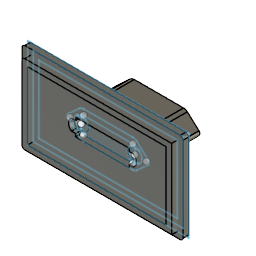
DD-fiche-v4 (Autodesk Fusion 360 design; units mm, degrees)
part number: 2025-12-20-11-26-56-309
Autodesk Fusion 360 part; units mm, degrees
note: some values were not read from the file. Set by a fixed rule: which sketch regions a step uses.
sketch "Esquisse1" plane through (0, 0, 0) normal (0, 1, 0) x (1, 0, 0)
  circle A0 centre (10, -10) radius 2.5
  line L0 (8.5, -12) -> (11.5, -12)
  line L1 (8.5, -8) -> (11.5, -8)
  circle A1 centre (29, -10) radius 2.5
  line L2 (27.5, -12) -> (30.5, -12)
  line L3 (27.5, -8) -> (30.5, -8)
  line L4 (5.3139, -10.7399) -> (9.4279, -14.4799)
  line L5 (10.7732, -15) -> (28.2268, -15)
  line L6 (29.5721, -14.4799) -> (33.6861, -10.7399)
  line L7 (33.6861, -9.2601) -> (29.5721, -5.5201)
  line L8 (28.2268, -5) -> (10.7732, -5)
  line L9 (9.4279, -5.5201) -> (5.3139, -9.2601)
  arc A2 (9.4279, -14.4799) -> (10.7732, -15) centre (10.7732, -13) ccw
  arc A3 (28.2268, -15) -> (29.5721, -14.4799) centre (28.2268, -13) ccw
  arc A4 (29.5721, -5.5201) -> (28.2268, -5) centre (28.2268, -7) ccw
  arc A5 (10.7732, -5) -> (9.4279, -5.5201) centre (10.7732, -7) ccw
  arc A6 (5.3139, -9.2601) -> (5.3139, -10.7399) centre (5.9866, -10) ccw
  arc A7 (33.6861, -10.7399) -> (33.6861, -9.2601) centre (33.0134, -10) ccw
  line L10 (-8.9501, 6) -> (48.0499, 6)
  line L11 (48.0499, 6) -> (48.0499, -26)
  line L12 (48.0499, -26) -> (-8.9501, -26)
  line L13 (-8.9501, -26) -> (-8.9501, 6)
  line L14 (-7, -24) -> (46, -24)
  line L15 (46, -24) -> (46, 4)
  line L16 (46, 4) -> (-7, 4)
  line L17 (-7, 4) -> (-7, -24)
  line L18 (-5, -22) -> (44, -22)
  line L19 (44, -22) -> (44, 2)
  line L20 (44, 2) -> (-5, 2)
  line L21 (-5, 2) -> (-5, -22)
  line L22 (10, -12) -> (8.5, -12)
  line L23 (10, -13) -> (29, -13)
  line L24 (29, -7) -> (10, -7)
  line L25 (10, -13) -> (10, -7)
  line L26 (29, -13) -> (29, -7)
  constraint coincident A0 L0.start
  constraint coincident A0 L0.end
  constraint horizontal L0
  constraint coincident A0 L1.start
  constraint coincident A0 L1.end
  constraint parallel L0 L1
  constraint coincident A1 L2.start
  constraint coincident A1 L2.end
  constraint horizontal L2
  constraint coincident A1 L3.start
  constraint coincident A1 L3.end
  constraint parallel L2 L3
  constraint horizontal L5
  constraint horizontal L8
  constraint equal A2 A3
  constraint equal A2 A4
  constraint equal A2 A5
  constraint horizontal L10
  constraint vertical L11
  constraint horizontal L12
  constraint vertical L13
  constraint horizontal L14
  constraint vertical L15
  constraint horizontal L16
  constraint vertical L17
  constraint horizontal L18
  constraint vertical L19
  constraint horizontal L20
  constraint vertical L21
  constraint midpoint L0 L22.start
  constraint parallel L3 L24
  constraint perpendicular L24 L25
  constraint perpendicular L24 L26
extrude "Extrusion23" add sketch "Esquisse1" against normal blind 2 contours A0 L1 L25 | A0 L0 L22 L25 | A1 L3 L26 | A1 L2 L26 | L4 L5 L6 L7 L8 L9 A2 A3 A4 A5 A6 A7 | L10 L11 L12 L13 | L14 L15 L16 L17 | L18 L19 L20 L21 picked at (9.893, -7.6736) picked at (29.107, -7.6736) picked at (29.107, -12.3264) makes body 1
extrude "Extrusion24" add sketch "Esquisse1" against normal blind 4 separate body contours L14 L15 L16 L17 makes body 2
extrude "Extrusion25" add sketch "Esquisse1" along normal blind 18 separate body contours A0 A1 L23 L24 L25 L26 | A0 L1 L25 | A0 L0 L25 | A0 L1 L25 | A0 L0 L22 L25 | A1 L3 L26 | A1 L3 L26 | A1 L2 L26 | A1 L2 L26 | L4 L5 L6 L7 L8 L9 A2 A3 A4 A5 A6 A7 makes body 3
extrude "Extrusion26" add sketch "Esquisse1" along normal blind 8 separate body contours A0 A1 L23 L24 L25 L26 makes body 4
extrude "Extrusion27" add sketch "Esquisse1" along normal blind 2 separate body contours A0 A1 L23 L24 L25 L26 makes body 5
fillet "Congé5" radius 1 1 edges at (-8.9501, -1, -6) on bodies 1
fillet "Congé6" radius 1 1 edges at (48.0499, -1, -6) on bodies 1
fillet "Congé7" radius 1 1 edges at (48.0499, -1, 26) on bodies 1
fillet "Congé8" radius 1 1 edges at (-8.9501, -1, 26) on bodies 1
fillet "Congé9" radius 1 1 edges at (-7, -2, -4) on bodies 2
fillet "Congé10" radius 1 1 edges at (-7, -2, 24) on bodies 2
